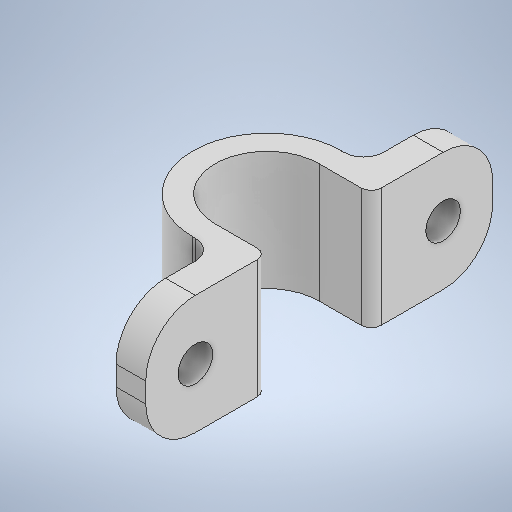
# Autodesk Inventor part: tube_holder
Saved by Autodesk Inventor 2025.2 (Build 292293000, 293)
## iProperties
Created: 2025-01-26
Part Number: tube_holder
Material: Типовые
Document SubType Name: Modeling
Designer: Admin
Density: 1 g/cm^3
Appearance: По умолчанию
Author: Admin
Autodesk Inventor part; units mm, degrees
ref_plane "YZ Plane" through (0, 0, 0) normal (1, 0, 0) x (0, 1, 0)
ref_plane "XZ Plane" through (0, 0, 0) normal (0, 1, 0) x (-1, 0, 0)
ref_plane "XY Plane" through (0, 0, 0) normal (0, 0, 1) x (1, 0, 0)
sketch "Эскиз1" plane through (0, 0, 0) normal (0, 1, 0) x (-1, 0, 0)
  arc A0 (0, -5.25) -> (0, 5.25) centre (0, 0) ccw
  arc A1 (0, -7.5) -> (0, 7.5) centre (0, 0) ccw
  line L0 (0, 7.5) -> (-0.25, 7.5)
  line L1 (-5.25, 6.25) -> (-5.25, 17.5)
  line L2 (-5.25, -17.5) -> (-5.25, -6.25)
  line L3 (-0.25, -7.5) -> (0, -7.5)
  line L4 (-5.25, 17.5) -> (-2.25, 17.5)
  line L5 (-2.25, 17.5) -> (-2.25, 9.5)
  line L6 (-2.25, -9.5) -> (-2.25, -17.5)
  line L7 (-2.25, -17.5) -> (-5.25, -17.5)
  line L8 (0, 5.25) -> (-4.25, 5.25)
  line L9 (0, -5.25) -> (-4.25, -5.25)
  arc A2 (-2.25, 9.5) -> (-0.25, 7.5) centre (-0.25, 9.5) ccw
  arc A3 (-0.25, -7.5) -> (-2.25, -9.5) centre (-0.25, -9.5) ccw
  arc A4 (-5.25, 6.25) -> (-4.25, 5.25) centre (-4.25, 6.25) ccw
  arc A5 (-4.25, -5.25) -> (-5.25, -6.25) centre (-4.25, -6.25) ccw
  point P0 (-2.25, -7.5)
  dimension "d0" = 10.5
  dimension "d4" = 3
  dimension "d5" = 2
  dimension "d6" = 1
  constraints: 20 end point, 12 point on circle, 12 tangent, 6 centre point, 5 point on line, 3 horizontal, 3 perpendicular, 2 coincident, 2 equal radius
  measures "d0" diameter of A0
  measures "d4" distance of L1.end L4.end
  measures "d5" radius of A2
  measures "d6" radius of A4
extrude "Выдавливание1" add sketch "Эскиз1" along normal blind 12
fillet "Сопряжение1" radius 5 4 edges at (3.75, 12, 17.5) (3.75, 0, 17.5) (3.75, 12, -17.5) (3.75, 0, -17.5)
sketch "Эскиз2" plane through (2.25, 0, 9.5) normal (-1, 0, 0) x (0, 0, 1)
  line L0 (8, 5) -> (8, 7) projected
  line L1 (8, 6) -> (3, 6)
  circle A0 centre (3, 6) radius 1.75
  line L2 (-27, 5) -> (-27, 7) projected
  line L3 (-27, 6) -> (-22, 6)
  circle A1 centre (-22, 6) radius 1.75
  point P0 (-9.5, 0)
  dimension "d10" = 5
  dimension "d11" = 3.5
  dimension "d12" = 5
  dimension "d13" = 3.5
  constraints: 4 end point, 2 centre point, 2 coincident, 2 horizontal, 2 midpoint
  measures "d10" distance of L1.start L1.end
  measures "d11" diameter of A0
  measures "d12" distance of L3.start L3.end
  measures "d13" diameter of A1
extrude "Выдавливание2" cut sketch "Эскиз2" against normal through all
